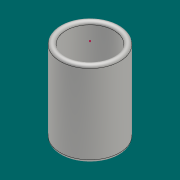
# Autodesk Inventor part: cup
Saved by Autodesk Inventor 2018 (Build 220112000, 112)
## iProperties
Created: 2021-12-25
Part Number: cup
Material: アルミニウム 6061
Document SubType Name: Modeling
Designer: gisen
Density: 2.7 g/cm^3
Appearance: アルミニウム - フラット
Author: gisen
Autodesk Inventor part; units mm, degrees
ref_plane "YZ Plane" through (0, 0, 0) normal (1, 0, 0) x (0, 1, 0)
ref_plane "XZ Plane" through (0, 0, 0) normal (0, 1, 0) x (-1, 0, 0)
ref_plane "XY Plane" through (0, 0, 0) normal (0, 0, 1) x (1, 0, 0)
sketch "スケッチ1" plane through (0, 0, 0) normal (0, 0, 1) x (1, 0, 0)
  line L0 (-45, 45) -> (45, 45)
  line L1 (45, 45) -> (45, -45)
  line L2 (45, -45) -> (-45, -45)
  line L3 (-45, -45) -> (-45, 45)
  point P0 (0, 0)
  point P1 (0, 45)
  point P2 (-45, 0)
  dimension "d0" = 90
  dimension "d1" = 90
  constraints: 8 end point, 2 midpoint, 2 parallel, 1 horizontal, 1 horizontal alignment, 1 perpendicular, 1 vertical alignment
  measures "d0" distance of L0.start L0.end
  measures "d1" distance of L2.end L0.start
extrude "押し出し1" add sketch "スケッチ1" along normal blind 180
sketch "スケッチ2" plane through (0, 0, 180) normal (0, 0, 1) x (1, 0, 0)
  point P0 (0, 0)
sketch "スケッチ3" plane through (0, 0, 180) normal (0, 0, 1) x (1, 0, 0)
  circle A0 centre (0, 0) radius 42
  dimension "d4" = 84
  constraints: 1 centre point, 1 coincident
  measures "d4" diameter of A0
extrude "押し出し2" cut sketch "スケッチ3" against normal through all keep common part
sketch "スケッチ4" plane through (0, 0, 180) normal (0, 0, 1) x (1, 0, 0)
  circle A0 centre (0, 0) radius 34
  circle A1 centre (0, 0) radius 42 construction
  dimension "d7" = 8
  constraints: 1 centre point, 1 coincident
  measures "d7" radial gap between concentric circles of A1 A0
extrude "押し出し3" cut sketch "スケッチ4" against normal blind 100
sketch "スケッチ5" plane through (0, 0, 0) normal (0, 0, -1) x (-1, 0, 0)
  circle A0 centre (0, 0) radius 42 projected
extrude "押し出し4" cut sketch "スケッチ5" against normal blind 60
fillet "フィレット1" radius 20 1 edges at (-34, 0, 80)
sketch "スケッチ6" plane through (0, 0, 60) normal (0, 0, -1) x (-1, 0, 0)
  circle A0 centre (0, 0) radius 34 projected
extrude "押し出し5" cut sketch "スケッチ6" against normal blind 8
fillet "フィレット2" radius 4 4 edges at (-42, 0, 180) (-34, 0, 180) (-42, 0, 60) (34, 0, 60)
fillet "フィレット3" radius 20 1 edges at (34, 0, 68)
equation "\"d1\" = d0"
